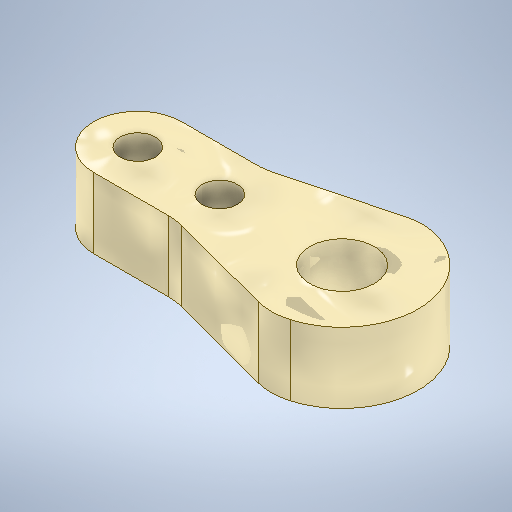
# Autodesk Inventor part: adaptator_25
Saved by Autodesk Inventor 2025 (Build 290162000, 162)
## iProperties
Created: 2024-12-10
Part Number: adaptator_25
Material: Generic
Document SubType Name: Modeling
Designer: Pauline Simonnet
Density: 1 g/cm^3
Appearance: Fine - Cream
Author: Pauline Simonnet
Autodesk Inventor part; units mm, degrees
ref_plane "YZ Plane" through (0, 0, 0) normal (1, 0, 0) x (0, 1, 0)
ref_plane "XZ Plane" through (0, 0, 0) normal (0, 1, 0) x (-1, 0, 0)
ref_plane "XY Plane" through (0, 0, 0) normal (0, 0, 1) x (1, 0, 0)
sketch "Sketch1" plane through (0, 0, 0) normal (0, 1, 0) x (-1, 0, 0)
  arc A0 (0, 6.5) -> (0, -6.5) centre (0, 0) ccw
  arc A1 (17.43, -3.75) -> (17.43, 3.75) centre (17.43, 0) ccw
  line L0 (10.43, 3.75) -> (17.43, 3.75)
  line L1 (10.43, -3.75) -> (17.43, -3.75)
  line L2 (0, 0) -> (20.86, 0) construction
  circle A2 centre (0, 0) radius 2.75
  circle A3 centre (17.43, 0) radius 1.5
  circle A4 centre (10.43, 0) radius 1.5
  line L3 (10.43, 3.75) -> (0, 6.5)
  line L4 (10.43, -3.75) -> (0, -6.5)
  line L5 (10.43, 0) -> (10.43, -12.3931) construction
  line L6 (0, 8.169) -> (0, -9.3531) construction
  dimension "d0" = 13
  dimension "d1" = 7.5
  dimension "d2" = 17.43
  dimension "d3" = 7.5
  dimension "d6" = 0
  dimension "d7" = 3.75
  dimension "d8" = 5.5
  dimension "d10" = 3
  dimension "d11" = 3
  dimension "d14" = 7
  dimension "d17" = 17.43
  dimension "d20" = 0
  dimension "d21" = 0
  dimension "d22" = 0
  dimension "d23" = 0
  dimension "d24" = 0
  constraints: 14 end point, 5 centre point, 4 point on circle, 3 horizontal, 2 coincident, 2 vertical, 1 midpoint, 1 point on line
  measures "d0" diameter of A0
  measures "d1" diameter of A1
  measures "d2" distance of point (0, 0) A1.centre
  measures "d3" distance between parallel lines of L1 L0
  measures "d6" distance from line of L2 A1.centre
  measures "d7" distance between parallel lines of L2 L0
  measures "d8" diameter of A2
  measures "d10" diameter of A4
  measures "d11" diameter of A3
  measures "d14" distance of L5.start A3.centre
  measures "d17" distance of point (0, 0) A3.centre
  measures "d20" distance from line of L5 L1.start
  measures "d21" distance from line of L5 L0.start
  measures "d22" distance from line of L6 L3.end
  measures "d23" distance from line of L6 L4.end
  measures "d24" distance from line of point (0, 0) L6
extrude "Extrusion1" add sketch "Sketch1" along normal blind 6
fillet "Fillet1" radius 5 1 edges at (-10.43, 3, 3.75)
fillet "Fillet2" radius 5 1 edges at (-10.43, 3, -3.75)
fillet "Fillet3" radius 5 2 edges at (0, 3, -6.5) (0, 3, 6.5)
body "Solid1"
